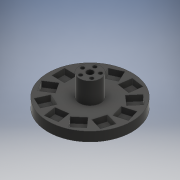
# Autodesk Inventor part: SG02
Saved by Autodesk Inventor 2017 (Build 210142000, 142)
## iProperties
Created: 2019-09-21
Part Number: SG02
Material: ABS Plastic
Document SubType Name: Modeling
Designer: Dell
Density: 1.06 g/cm^3
Appearance: Smooth - Black
Author: Dell
Autodesk Inventor part; units mm, degrees
ref_plane "YZ Plane" through (0, 0, 0) normal (1, 0, 0) x (0, 1, 0)
ref_plane "XZ Plane" through (0, 0, 0) normal (0, 1, 0) x (-1, 0, 0)
ref_plane "XY Plane" through (0, 0, 0) normal (0, 0, 1) x (1, 0, 0)
sketch "Sketch2" plane through (0, 0, 0) normal (0, 0, 1) x (1, 0, 0)
  circle A0 centre (0, 0) radius 45
  dimension "d0" = 90
  constraints: 1 centre point, 1 coincident
  measures "d0" diameter of A0
extrude "Extrusion1" add sketch "Sketch2" along normal blind 10
sketch "Sketch4" plane through (0, 0, 10) normal (0, 0, 1) x (1, 0, 0)
  circle A0 centre (0, 0) radius 11.5
  dimension "d14" = 23
  constraints: 1 centre point, 1 coincident
  measures "d14" diameter of A0
extrude "Extrusion3" add sketch "Sketch4" along normal blind 23
sketch "Sketch5" plane through (0, 0, 33) normal (0, 0, 1) x (1, 0, 0)
  circle A0 centre (-8, 0) radius 2
  circle A1 centre (0, 0) radius 3.5
  circle A2 centre (0, 0) radius 11.5 construction
  circle A3 centre (-2.4721, -7.6085) radius 2
  circle A4 centre (6.4721, -4.7023) radius 2
  circle A5 centre (6.4721, 4.7023) radius 2
  circle A6 centre (-2.4721, 7.6085) radius 2
  dimension "d19" = 4
  dimension "d20" = 8
  dimension "d21" = 360
  dimension "d22" = 7
  constraints: 7 centre point, 1 coincident, 1 horizontal alignment, 11 other
  measures "d19" diameter of A0
  measures "d20" distance of point (0, 0) A0.centre
  measures "d22" diameter of A1
extrude "Extrusion4" cut sketch "Sketch5" against normal through all
sketch "Sketch6" plane through (0, 0, 10) normal (0, 0, 1) x (1, 0, 0)
  line L0 (-40, 0) -> (-27.3, 0)
  line L1 (-27.3, 0) -> (-27.3, 12.7)
  line L2 (-27.3, 12.7) -> (-40, 12.7)
  line L3 (-40, 12.7) -> (-40, 0)
  line L4 (-40.5, 13.2) -> (-26.8, 13.2)
  line L5 (-26.8, 13.2) -> (-26.8, -0.5)
  line L6 (-26.8, -0.5) -> (-40.5, -0.5)
  line L7 (-40.5, -0.5) -> (-40.5, 13.2)
  line L8 (-33.6501, -21.6256) -> (-22.9662, -14.7595)
  line L9 (-22.9662, -14.7595) -> (-29.8324, -4.0756)
  line L10 (-29.8324, -4.0756) -> (-40.5163, -10.9417)
  line L11 (-40.5163, -10.9417) -> (-33.6501, -21.6256)
  line L12 (-41.2072, -10.7914) -> (-29.6821, -3.3846)
  line L13 (-29.6821, -3.3846) -> (-22.2753, -14.9098)
  line L14 (-22.2753, -14.9098) -> (-33.8004, -22.3166)
  line L15 (-33.8004, -22.3166) -> (-41.2072, -10.7914)
  line L16 (-16.6166, -36.3853) -> (-11.3408, -24.833)
  line L17 (-11.3408, -24.833) -> (-22.8932, -19.5572)
  line L18 (-22.8932, -19.5572) -> (-28.1689, -31.1095)
  line L19 (-28.1689, -31.1095) -> (-16.6166, -36.3853)
  line L20 (-28.8315, -31.3566) -> (-23.1403, -18.8947)
  line L21 (-23.1403, -18.8947) -> (-10.6783, -24.5858)
  line L22 (-10.6783, -24.5858) -> (-16.3695, -37.0478)
  line L23 (-16.3695, -37.0478) -> (-28.8315, -31.3566)
  line L24 (5.6926, -39.5929) -> (3.8852, -27.0221)
  line L25 (3.8852, -27.0221) -> (-8.6855, -28.8295)
  line L26 (-8.6855, -28.8295) -> (-6.8781, -41.4003)
  line L27 (-6.8781, -41.4003) -> (5.6926, -39.5929)
  line L28 (-7.3019, -41.9663) -> (-9.2516, -28.4058)
  line L29 (-9.2516, -28.4058) -> (4.3089, -26.4561)
  line L30 (4.3089, -26.4561) -> (6.2587, -40.0166)
  line L31 (6.2587, -40.0166) -> (-7.3019, -41.9663)
  line L32 (26.1944, -30.23) -> (17.8777, -20.632)
  line L33 (17.8777, -20.632) -> (8.2797, -28.9487)
  line L34 (8.2797, -28.9487) -> (16.5964, -38.5467)
  line L35 (16.5964, -38.5467) -> (26.1944, -30.23)
  line L36 (16.546, -39.252) -> (7.5744, -28.8983)
  line L37 (7.5744, -28.8983) -> (17.9281, -19.9267)
  line L38 (17.9281, -19.9267) -> (26.8997, -30.2804)
  line L39 (26.8997, -30.2804) -> (16.546, -39.252)
  line L40 (38.3797, -11.2693) -> (26.1942, -7.6913)
  line L41 (26.1942, -7.6913) -> (22.6162, -19.8769)
  line L42 (22.6162, -19.8769) -> (34.8017, -23.4549)
  line L43 (34.8017, -23.4549) -> (38.3797, -11.2693)
  line L44 (35.1406, -24.0755) -> (21.9955, -20.2157)
  line L45 (21.9955, -20.2157) -> (25.8553, -7.0707)
  line L46 (25.8553, -7.0707) -> (39.0003, -10.9304)
  line L47 (39.0003, -10.9304) -> (35.1406, -24.0755)
  line L48 (38.3797, 11.2693) -> (26.1942, 7.6913)
  line L49 (26.1942, 7.6913) -> (29.7722, -4.4943)
  line L50 (29.7722, -4.4943) -> (41.9577, -0.9163)
  line L51 (41.9577, -0.9163) -> (38.3797, 11.2693)
  line L52 (42.5783, -1.2551) -> (29.4333, -5.1149)
  line L53 (29.4333, -5.1149) -> (25.5735, 8.0302)
  line L54 (25.5735, 8.0302) -> (38.7186, 11.8899)
  line L55 (38.7186, 11.8899) -> (42.5783, -1.2551)
  line L56 (26.1944, 30.23) -> (17.8777, 20.632)
  line L57 (17.8777, 20.632) -> (27.4757, 12.3152)
  line L58 (27.4757, 12.3152) -> (35.7924, 21.9133)
  line L59 (35.7924, 21.9133) -> (26.1944, 30.23)
  line L60 (36.4978, 21.9637) -> (27.5262, 11.6099)
  line L61 (27.5262, 11.6099) -> (17.1724, 20.5815)
  line L62 (17.1724, 20.5815) -> (26.144, 30.9353)
  line L63 (26.144, 30.9353) -> (36.4978, 21.9637)
  line L64 (5.6926, 39.5929) -> (3.8852, 27.0221)
  line L65 (3.8852, 27.0221) -> (16.4559, 25.2147)
  line L66 (16.4559, 25.2147) -> (18.2633, 37.7855)
  line L67 (18.2633, 37.7855) -> (5.6926, 39.5929)
  line L68 (18.8294, 38.2092) -> (16.8797, 24.6487)
  line L69 (16.8797, 24.6487) -> (3.3191, 26.5984)
  line L70 (3.3191, 26.5984) -> (5.2688, 40.1589)
  line L71 (5.2688, 40.1589) -> (18.8294, 38.2092)
  line L72 (-16.6166, 36.3853) -> (-11.3408, 24.833)
  line L73 (-11.3408, 24.833) -> (0.2115, 30.1087)
  line L74 (0.2115, 30.1087) -> (-5.0643, 41.6611)
  line L75 (-5.0643, 41.6611) -> (-16.6166, 36.3853)
  line L76 (-4.8172, 42.3236) -> (0.874, 29.8616)
  line L77 (0.874, 29.8616) -> (-11.5879, 24.1704)
  line L78 (-11.5879, 24.1704) -> (-17.2791, 36.6324)
  line L79 (-17.2791, 36.6324) -> (-4.8172, 42.3236)
  line L80 (-33.6501, 21.6256) -> (-22.9662, 14.7595)
  line L81 (-22.9662, 14.7595) -> (-16.1001, 25.4434)
  line L82 (-16.1001, 25.4434) -> (-26.784, 32.3096)
  line L83 (-26.784, 32.3096) -> (-33.6501, 21.6256)
  line L84 (-26.9343, 33.0005) -> (-15.4091, 25.5937)
  line L85 (-15.4091, 25.5937) -> (-22.8159, 14.0685)
  line L86 (-22.8159, 14.0685) -> (-34.3411, 21.4753)
  line L87 (-34.3411, 21.4753) -> (-26.9343, 33.0005)
  point P0 (0, 0)
  dimension "d25" = 12.7
  dimension "d26" = 12.7
  dimension "d27" = 40
  dimension "d28" = 0.5
  dimension "d31" = 360
  constraints: 176 end point, 4 parallel, 2 perpendicular, 1 horizontal, 1 horizontal alignment, 180 other
  measures "d25" distance of L2.end L1.end
  measures "d26" distance of L1.end L0.end
  measures "d27" distance of point (0, 0) L0.start
  measures "d28" distance between parallel lines of L2 L4
extrude "Extrusion5" cut sketch "Sketch6" against normal blind 6.35 contours L3 L2 L1 L0 | L4 L5 L6 L7 | L11 L10 L9 L8 | L12 L13 L14 L15 | L19 L18 L17 L16 | L20 L21 L22 L23 | L27 L26 L25 L24 | L28 L29 L30 L31 | L35 L34 L33 L32 | L36 L37 L38 L39 | L43 L42 L41 L40 | L44 L45 L46 L47 | L51 L50 L49 L48 | L52 L53 L54 L55 | L59 L58 L57 L56 | L60 L61 L62 L63 | L67 L66 L65 L64 | L68 L69 L70 L71 | L75 L74 L73 L72 | L76 L77 L78 L79 | L83 L82 L81 L80 | L84 L85 L86 L87
body "Solid1"
